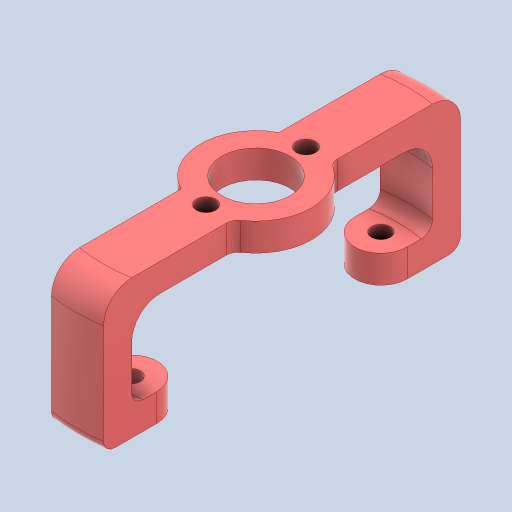
# Autodesk Inventor part: Th_3D_hn_2
Saved by Autodesk Inventor 2024 (Build 280153000, 153)
## iProperties
Created: 2020-11-15
Part Number: Th_3D_hn_2
Material: ABS プラスチック
Document SubType Name: Modeling
Designer: Haruka
Density: 1.06 g/cm^3
Appearance: 滑らか - 赤
Author: Haruka
Autodesk Inventor part; units mm, degrees
ref_plane "YZ Plane" through (0, 0, 0) normal (1, 0, 0) x (0, 1, 0)
ref_plane "XZ Plane" through (0, 0, 0) normal (0, 1, 0) x (-1, 0, 0)
ref_plane "XY Plane" through (0, 0, 0) normal (0, 0, 1) x (1, 0, 0)
sketch "スケッチ1" plane through (0, 0, 0) normal (0, 1, 0) x (-1, 0, 0)
  line L0 (0, 0) -> (0, -22.5) construction
  line L1 (0, 0) -> (0, 22.5) construction
  circle A0 centre (0, 22.5) radius 1.7
  circle A1 centre (0, -22.5) radius 1.7
  circle A2 centre (0, 22.5) radius 4.7
  circle A3 centre (0, -22.5) radius 4.7
  line L2 (4.6978, 32.1587) -> (4.7004, -32.1583)
  line L3 (-4.6974, 32.1587) -> (-4.6974, -32.1587)
  circle A4 centre (0, 0) radius 32.5
  point P0 (4.6982, 22.3711)
  point P1 (4.7, -22.4998)
  point P2 (-4.6974, 22.343)
  point P3 (-4.6974, -22.657)
  point P4 (-4.6974, 14.2455)
  point P5 (4.6986, 14.2451)
  point P6 (4.6997, -14.2448)
  point P7 (-4.6974, -14.2455)
  point P8 (4.6982, 22.6293)
  point P9 (-4.6974, 22.657)
  point P10 (4.7, -22.5)
  point P11 (-4.6974, -22.343)
  dimension "d0" = 22.5
  dimension "d1" = 22.5
  dimension "d2" = 3.4
  dimension "d3" = 3.4
  dimension "d5" = 3
  dimension "d6" = 3
  dimension "d7" = 65
  constraints: 8 end point, 8 point on circle, 5 centre point, 4 point on line, 3 coincident, 3 vertical, 1 tangent
  measures "d0" distance of L0.start L0.end
  measures "d1" distance of L0.start L1.end
  measures "d2" diameter of A0
  measures "d3" diameter of A1
  measures "d5" radial gap between concentric circles of A0 A2
  measures "d6" radial gap between concentric circles of A3 A1
  measures "d7" diameter of A4
extrude "押し出し1" add sketch "スケッチ1" along normal blind 5 contours A2 L3 | A2 L3 A4 L2 | L3 A2 | A3 L3 | L2 A4 L3 A3 | L3 A3
sketch "スケッチ2" plane through (0, 5, 0) normal (0, 1, 0) x (1, 0, 0)
  arc A0 (4.6974, -22.657) -> (-4.6982, -22.6293) centre (0, -22.5) ccw projected
  circle A1 centre (0, -22.5) radius 1.7 projected
  arc A2 (-4.7, 22.5) -> (4.6974, 22.657) centre (0, 22.5) ccw projected
  circle A3 centre (0, 22.5) radius 1.7 projected
  circle A4 centre (0, 0) radius 27.5
  line L0 (4.6974, 22.657) -> (4.6974, 32.1587) projected
  arc A5 (4.6974, 32.1587) -> (-4.7004, 32.1583) centre (0, 0) ccw projected
  line L1 (-4.7004, 32.1583) -> (-4.7, 22.5) projected
  line L2 (-4.6982, -22.6293) -> (-4.6978, -32.1587) projected
  arc A6 (-4.6978, -32.1587) -> (4.6974, -32.1587) centre (0, 0) ccw projected
  line L3 (4.6974, -32.1587) -> (4.6974, -22.657) projected
  point P0 (-4.7002, 27.0954)
  point P1 (4.6974, 27.0958)
  point P2 (4.6974, -27.0958)
  point P3 (-4.698, -27.0957)
  dimension "d10" = 55
  constraints: 1 centre point
  measures "d10" diameter of A4
extrude "押し出し2" add sketch "スケッチ2" along normal blind 15 contours L3 A6 L2 A4 | L1 A5 L0 A4
sketch "スケッチ3" plane through (0, 20, 0) normal (0, 1, 0) x (1, 0, 0)
  arc A0 (4.6974, 27.0958) -> (-4.7002, 27.0954) centre (0, 0) ccw projected
  arc A1 (-4.698, -27.0957) -> (4.6974, -27.0958) centre (0, 0) ccw projected
  line L0 (-4.698, -27.0957) -> (-4.698, 32.1586)
  line L1 (4.6974, -27.0958) -> (4.6974, 27.0958)
  circle A2 centre (0, 0) radius 10
  line L2 (4.6974, -32.1587) -> (4.6974, -27.0958) projected
  line L3 (-4.698, -27.0957) -> (-4.6978, -32.1587) projected
  arc A3 (-4.6978, -32.1587) -> (4.6974, -32.1587) centre (0, 0) ccw projected
  line L4 (-4.7004, 32.1583) -> (-4.7002, 27.0954) projected
  line L5 (4.6974, 27.0958) -> (4.6974, 32.1587) projected
  arc A4 (4.6974, 32.1587) -> (-4.7004, 32.1583) centre (0, 0) ccw projected
  line L6 (4.6974, -32.1587) -> (4.6974, -27.0958) projected
  arc A5 (-4.698, -27.0957) -> (4.6974, -27.0958) centre (0, 0) ccw projected
  line L7 (-4.698, -27.0957) -> (-4.6978, -32.1587) projected
  arc A6 (-4.6978, -32.1587) -> (4.6974, -32.1587) centre (0, 0) ccw projected
  point P0 (-4.698, 8.8277)
  point P1 (-4.698, -8.8277)
  point P2 (4.6974, -8.8281)
  point P3 (4.6974, 8.8281)
  point P4 (4.6974, -27.0958)
  dimension "d16" = 20
  constraints: 4 end point, 4 point on circle, 1 centre point, 1 coincident, 1 vertical
  measures "d16" diameter of A2
extrude "押し出し3" add sketch "スケッチ3" along normal blind 5 contours L1 A2 L0 A0 | A0 L0 A4 L5 | A2 L1 | L1 A2 L0 | L0 A2 | L1 A1 L0 A2 | L2 A3 L3 A1
sketch "スケッチ5" plane through (0, 25, 0) normal (0, 1, 0) x (1, 0, 0)
  circle A0 centre (0, 0) radius 6
  line L0 (0, 0) -> (0, 9)
  line L1 (0, 9) -> (0, -9)
  dimension "d18" = 12
  dimension "d19" = 9
  dimension "d20" = 18
  constraints: 4 coincident, 4 end point, 1 centre point, 1 point on line, 1 vertical
  measures "d18" diameter of A0
  measures "d19" distance of L0.start L0.end
  measures "d20" distance of L0.end L1.end
hole "穴1" at (0, 25, -9) at (0, 25, 9) direction (0, -1, 0) diameter 3.5 end through all
sketch "スケッチ6" plane through (0, 25, 0) normal (0, 1, 0) x (1, 0, 0)
  point P0 (0, 0)
  point P1 (0, 0)
  constraints: 1 coincident
hole "穴2" at (0, 25, 0) direction (0, -1, 0) diameter 12.35 end through all
fillet "フィレット3" radius 2 2 edges at (4.6974, 22.5, -8.8281) (4.6974, 22.5, 8.8281)
fillet "フィレット4" radius 2 4 edges at (-0.0015, 0, -32.5) (-0.0002, 0, 32.5) (-0.0003, 5, 27.5) (-0.0014, 5, -27.5)
fillet "フィレット5" radius 5 4 edges at (-0.0003, 20, 27.5) (-0.0003, 20, -27.5) (-0.0002, 25, 32.5) (-0.0003, 25, -32.5)
equation "\"d1\" = d0"
